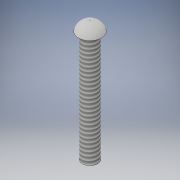
# Autodesk Inventor part: 0.156screw
Saved by Autodesk Inventor 2017 (Build 210142000, 142)
## iProperties
Created: 2019-02-05
Part Number: 0.156screw
Material: Generic
Document SubType Name: Modeling
Designer: S346559073
Density: 1 g/cm^3
Appearance: Default
Author: S346559073
Autodesk Inventor part; units mm, degrees
ref_plane "YZ Plane" through (0, 0, 0) normal (1, 0, 0) x (0, 1, 0)
ref_plane "XZ Plane" through (0, 0, 0) normal (0, 1, 0) x (-1, 0, 0)
ref_plane "XY Plane" through (0, 0, 0) normal (0, 0, 1) x (1, 0, 0)
sketch "Sketch1" plane through (0, 0, 0) normal (0, 1, 0) x (-1, 0, 0)
  circle A0 centre (0, 0) radius 2.0955
  dimension "d0" = 4.191
  constraints: 1 centre point, 1 coincident
  measures "d0" diameter of A0
extrude "Extrusion1" add sketch "Sketch1" along normal blind 30.48
sketch "Sketch2" plane through (0, 30.48, 0) normal (0, 1, 0) x (1, 0, 0)
  circle A0 centre (0, 0) radius 3.175
  dimension "d3" = 6.35
  constraints: 1 centre point, 1 coincident
  measures "d3" diameter of A0
extrude "Extrusion2" add sketch "Sketch2" along normal blind 2.54
fillet "Fillet1" radius 3.175 1 edges at (-3.175, 33.02, 0)
thread "Thread1" size "10-24 UNC" class "2A" standard "ANSI Unified Screw Threads" full length
body "Solid1"
